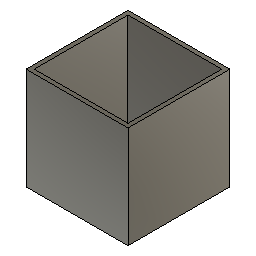
Calibration-Box (Autodesk Fusion 360 design; units mm, degrees)
Autodesk Fusion 360 part; units mm, degrees
sketch "Sketch1" plane through (0, 0, 0) normal (0, 1, 0) x (1, 0, 0)
  line L0 (10, 10) -> (-10, 10)
  line L1 (-10, 10) -> (-10, -10)
  line L2 (-10, -10) -> (10, -10)
  line L3 (10, -10) -> (10, 10)
  line L4 (10, 10) -> (-10, -10) construction
  line L5 (-10, 10) -> (10, -10) construction
  dimension "d1" = 20
  dimension "d2" = 20
  constraint horizontal L0
  constraint perpendicular L0 L1
  constraint parallel L0 L2
  constraint parallel L1 L3
  constraint coincident L4 origin
  constraint coincident L5 origin
  measures "d1" distance of L0.start L0.end
  measures "d2" distance of L0.end L1.end
extrude "Extrude1" add sketch "Sketch1" along normal blind 20
sketch "Sketch2" plane through (0, 0, 10) normal (0, 0, 1) x (-1, 0, 0)
  line L0 (10, 0) -> (-10, 0)
  line L1 (-10, 0) -> (-10, -20)
  line L2 (-10, -20) -> (10, -20)
  line L3 (10, -20) -> (10, 0)
  line L4 (9.2, -0.8) -> (9.2, -19.2)
  line L5 (9.2, -19.2) -> (-9.2, -19.2)
  line L6 (-9.2, -19.2) -> (-9.2, -0.8)
  line L7 (-9.2, -0.8) -> (9.2, -0.8)
  dimension "d5" = 0.8
  dimension "d6" = 0.8
  dimension "d7" = 0.8
  dimension "d8" = 0.8
  constraint vertical L4
  constraint perpendicular L4 L5
  constraint perpendicular L5 L6
  constraint perpendicular L4 L7
  measures "d5" distance of L0 L7
  measures "d6" distance of L3 L4
  measures "d7" distance of L2 L5
  measures "d8" distance of L1 L6
extrude "Extrude2" cut sketch "Sketch2" against normal blind 19.2 contours L4 L5 L6 L7
